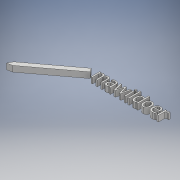
# Autodesk Inventor part: Matt
Saved by Autodesk Inventor 2017 (Build 210142000, 142)
## iProperties
Created: 2021-02-26
Part Number: Matt
Material: Generic
Document SubType Name: Modeling
Designer: paulg
Density: 1 g/cm^3
Appearance: Default
Author: paulg
Autodesk Inventor part; units mm, degrees
ref_plane "YZ Plane" through (0, 0, 0) normal (1, 0, 0) x (0, 1, 0)
ref_plane "XZ Plane" through (0, 0, 0) normal (0, 1, 0) x (-1, 0, 0)
ref_plane "XY Plane" through (0, 0, 0) normal (0, 0, 1) x (1, 0, 0)
sketch "Sketch1" plane through (0, 0, 0) normal (0, 0, 1) x (1, 0, 0)
  line L0 (-0.0217, 0.1086) -> (95.9171, 0.1086) construction
  line L1 (95.9171, 0.1086) -> (95.9171, -3.6211) construction
  line L2 (95.9171, -3.6211) -> (-0.0217, -3.6211) construction
  line L3 (-0.0217, -3.6211) -> (-0.0217, 0.1086) construction
  line L4 (-41.7116, -36.1087) -> (-2.9577, -7.16)
  line L5 (-2.9577, -7.16) -> (-5.3043, -4.0186)
  line L6 (-5.3043, -4.0186) -> (-44.0582, -32.9673)
  line L7 (-44.0582, -32.9673) -> (-41.7116, -36.1087)
  line L8 (-41.7116, -36.1087) -> (-5.3043, -4.0186) construction
  line L9 (-2.9577, -7.16) -> (-44.0582, -32.9673) construction
  line L10 (-44.0582, -32.9673) -> (-46.1916, -37.008)
  line L11 (-46.1916, -37.008) -> (-41.7116, -36.1087)
  line L12 (-46.1916, -37.008) -> (-42.8849, -34.538) construction
  line L13 (9.4029, -10.3371) -> (9.4029, -5.9935)
  spline S0 degree 2 poles (9.4029, -5.9935) (9.4029, -5.4748) (9.3219, -4.5915) (9.1922, -4.3484) knots 0 0 0 1 2 2 2
  spline S1 degree 2 poles (9.1922, -4.3484) (9.0625, -4.081) (8.5682, -3.8217) (8.1387, -3.8217) knots 0 0 0 1 2 2 2
  spline S2 degree 2 poles (8.1387, -3.8217) (7.7497, -3.8217) (6.8583, -4.2998) (6.3883, -4.7536) knots 0 0 0 1 2 2 2
  spline S3 degree 2 poles (6.3883, -4.7536) (6.3964, -4.867) (6.4126, -5.1831) (6.4126, -5.3938) knots 0 0 0 1 2 2 2
  line L14 (6.4126, -5.3938) -> (6.4126, -10.3371)
  line L15 (6.4126, -10.3371) -> (5.1484, -10.3371)
  line L16 (5.1484, -10.3371) -> (5.1484, -5.9935)
  spline S4 degree 2 poles (5.1484, -5.9935) (5.1484, -5.4748) (5.0674, -4.5915) (4.9378, -4.3484) knots 0 0 0 1 2 2 2
  spline S5 degree 2 poles (4.9378, -4.3484) (4.8081, -4.081) (4.3138, -3.8217) (3.8843, -3.8217) knots 0 0 0 1 2 2 2
  spline S6 degree 2 poles (3.8843, -3.8217) (3.4791, -3.8217) (2.5796, -4.3322) (2.1582, -4.7293) knots 0 0 0 1 2 2 2
  line L17 (2.1582, -4.7293) -> (2.1582, -10.3371)
  line L18 (2.1582, -10.3371) -> (0.894, -10.3371)
  line L19 (0.894, -10.3371) -> (0.894, -2.833)
  line L20 (0.894, -2.833) -> (2.1582, -2.833)
  line L21 (2.1582, -2.833) -> (2.1582, -3.6596)
  spline S7 degree 2 poles (2.1582, -3.6596) (2.6525, -3.1653) (3.6249, -2.6223) (4.2084, -2.6223) knots 0 0 0 1 2 2 2
  spline S8 degree 2 poles (4.2084, -2.6223) (4.8729, -2.6223) (5.9021, -3.2301) (6.1695, -3.9189) knots 0 0 0 1 2 2 2
  spline S9 degree 2 poles (6.1695, -3.9189) (6.7449, -3.2787) (7.8308, -2.6223) (8.4629, -2.6223) knots 0 0 0 1 2 2 2
  spline S10 degree 2 poles (8.4629, -2.6223) (8.9491, -2.6223) (9.7433, -2.9221) (10.035, -3.2625) knots 0 0 0 1 2 2 2
  spline S11 degree 2 poles (10.035, -3.2625) (10.3348, -3.6029) (10.6671, -4.6239) (10.6671, -5.3938) knots 0 0 0 1 2 2 2
  line L22 (10.6671, -5.3938) -> (10.6671, -10.3371)
  line L23 (10.6671, -10.3371) -> (9.4029, -10.3371)
  spline S12 degree 2 poles (16.6233, -9.5429) (16.4694, -9.6563) (15.9507, -10.0615) (15.7076, -10.1831) knots 0 0 0 1 2 2 2
  spline S13 degree 2 poles (15.7076, -10.1831) (15.3754, -10.3614) (14.7514, -10.5478) (14.1841, -10.5478) knots 0 0 0 1 2 2 2
  spline S14 degree 2 poles (14.1841, -10.5478) (13.7222, -10.5478) (12.8875, -10.1993) (12.5715, -9.8833) knots 0 0 0 1 2 2 2
  spline S15 degree 2 poles (12.5715, -9.8833) (12.2716, -9.5753) (11.907, -8.6677) (11.907, -8.1653) knots 0 0 0 1 2 2 2
  spline S16 degree 2 poles (11.907, -8.1653) (11.907, -7.3873) (12.5634, -6.2852) (13.2765, -5.9692) knots 0 0 0 1 2 2 2
  spline S17 degree 2 poles (13.2765, -5.9692) (13.9086, -5.6774) (15.6266, -5.4586) (16.6233, -5.4019) knots 0 0 0 1 2 2 2
  line L24 (16.6233, -5.4019) -> (16.6233, -5.1588)
  spline S18 degree 2 poles (16.6233, -5.1588) (16.6233, -4.7212) (16.3559, -4.1782) (16.1128, -4.0243) knots 0 0 0 1 2 2 2
  spline S19 degree 2 poles (16.1128, -4.0243) (15.8697, -3.8703) (15.1728, -3.773) (14.8, -3.773) knots 0 0 0 1 2 2 2
  spline S20 degree 2 poles (14.8, -3.773) (14.3624, -3.773) (13.1792, -4.0324) (12.5877, -4.2836) knots 0 0 0 1 2 2 2
  line L25 (12.5877, -4.2836) -> (12.5147, -4.2836)
  line L26 (12.5147, -4.2836) -> (12.5147, -2.9951)
  spline S21 degree 2 poles (12.5147, -2.9951) (12.8632, -2.8978) (14.1679, -2.6547) (14.8081, -2.6547) knots 0 0 0 1 2 2 2
  spline S22 degree 2 poles (14.8081, -2.6547) (15.5861, -2.6547) (16.6476, -2.8978) (17.069, -3.2139) knots 0 0 0 1 2 2 2
  spline S23 degree 2 poles (17.069, -3.2139) (17.4823, -3.5218) (17.8875, -4.5024) (17.8875, -5.2074) knots 0 0 0 1 2 2 2
  line L27 (17.8875, -5.2074) -> (17.8875, -10.3371)
  line L28 (17.8875, -10.3371) -> (16.6233, -10.3371)
  line L29 (16.6233, -10.3371) -> (16.6233, -9.5429)
  line L30 (16.6233, -8.4894) -> (16.6233, -6.4068)
  spline S24 degree 2 poles (16.6233, -6.4068) (16.1695, -6.4473) (14.8, -6.585) (14.3705, -6.7147) knots 0 0 0 1 2 2 2
  spline S25 degree 2 poles (14.3705, -6.7147) (13.8681, -6.8687) (13.2117, -7.5089) (13.2117, -8.0761) knots 0 0 0 1 2 2 2
  spline S26 degree 2 poles (13.2117, -8.0761) (13.2117, -8.7244) (13.941, -9.3808) (14.6379, -9.3808) knots 0 0 0 1 2 2 2
  spline S27 degree 2 poles (14.6379, -9.3808) (15.2295, -9.3808) (16.2019, -8.8703) (16.6233, -8.4894) knots 0 0 0 1 2 2 2
  line L31 (28.7546, -2.833) -> (26.8502, -10.3371)
  line L32 (26.8502, -10.3371) -> (25.6833, -10.3371)
  line L33 (25.6833, -10.3371) -> (23.8519, -4.551)
  line L34 (23.8519, -4.551) -> (22.0285, -10.3371)
  line L35 (22.0285, -10.3371) -> (20.8697, -10.3371)
  line L36 (20.8697, -10.3371) -> (18.9491, -2.833)
  line L37 (18.9491, -2.833) -> (20.2619, -2.833)
  line L38 (20.2619, -2.833) -> (21.5909, -8.6434)
  line L39 (21.5909, -8.6434) -> (23.3656, -2.833)
  line L40 (23.3656, -2.833) -> (24.411, -2.833)
  line L41 (24.411, -2.833) -> (26.2343, -8.6434)
  line L42 (26.2343, -8.6434) -> (27.4823, -2.833)
  line L43 (27.4823, -2.833) -> (28.7546, -2.833)
  line L44 (31.1533, -10.3371) -> (29.8891, -10.3371)
  line L45 (29.8891, -10.3371) -> (29.8891, -2.833)
  line L46 (29.8891, -2.833) -> (31.1533, -2.833)
  line L47 (31.1533, -2.833) -> (31.1533, -10.3371)
  line L48 (31.2425, -1.585) -> (29.8081, -1.585)
  line L49 (29.8081, -1.585) -> (29.8081, -0.2722)
  line L50 (29.8081, -0.2722) -> (31.2425, -0.2722)
  line L51 (31.2425, -0.2722) -> (31.2425, -1.585)
  line L52 (34.2976, -10.3371) -> (33.0334, -10.3371)
  line L53 (33.0334, -10.3371) -> (33.0334, 0.1086)
  line L54 (33.0334, 0.1086) -> (34.2976, 0.1086)
  line L55 (34.2976, 0.1086) -> (34.2976, -10.3371)
  line L56 (41.9232, -10.3371) -> (40.659, -10.3371)
  line L57 (40.659, -10.3371) -> (40.659, -9.5753)
  spline S28 degree 2 poles (40.659, -9.5753) (40.3672, -9.8184) (39.9378, -10.1426) (39.646, -10.2803) knots 0 0 0 1 2 2 2
  spline S29 degree 2 poles (39.646, -10.2803) (39.3786, -10.41) (38.8032, -10.5478) (38.4224, -10.5478) knots 0 0 0 1 2 2 2
  spline S30 degree 2 poles (38.4224, -10.5478) (37.8065, -10.5478) (36.7692, -10.0372) (36.4045, -9.5429) knots 0 0 0 1 2 2 2
  spline S31 degree 2 poles (36.4045, -9.5429) (36.0399, -9.0486) (35.6347, -7.5899) (35.6347, -6.6418) knots 0 0 0 1 2 2 2
  spline S32 degree 2 poles (35.6347, -6.6418) (35.6347, -5.6531) (36.1452, -4.2106) (36.5909, -3.6677) knots 0 0 0 1 2 2 2
  spline S33 degree 2 poles (36.5909, -3.6677) (37.0042, -3.1815) (38.163, -2.6223) (38.8032, -2.6223) knots 0 0 0 1 2 2 2
  spline S34 degree 2 poles (38.8032, -2.6223) (39.3624, -2.6223) (40.1971, -2.8735) (40.659, -3.1328) knots 0 0 0 1 2 2 2
  line L58 (40.659, -3.1328) -> (40.659, 0.1086)
  line L59 (40.659, 0.1086) -> (41.9232, 0.1086)
  line L60 (41.9232, 0.1086) -> (41.9232, -10.3371)
  line L61 (40.659, -8.5137) -> (40.659, -4.1782)
  spline S35 degree 2 poles (40.659, -4.1782) (40.189, -3.9513) (39.4434, -3.7811) (39.0139, -3.7811) knots 0 0 0 1 2 2 2
  spline S36 degree 2 poles (39.0139, -3.7811) (38.0415, -3.7811) (36.9394, -5.2398) (36.9394, -6.6174) knots 0 0 0 1 2 2 2
  spline S37 degree 2 poles (36.9394, -6.6174) (36.9394, -7.9465) (37.7822, -9.3484) (38.7141, -9.3484) knots 0 0 0 1 2 2 2
  spline S38 degree 2 poles (38.7141, -9.3484) (39.2084, -9.3484) (40.2133, -8.8946) (40.659, -8.5137) knots 0 0 0 1 2 2 2
  spline S39 degree 2 poles (49.9215, -6.585) (49.9215, -8.4813) (48.0982, -10.5478) (46.5747, -10.5478) knots 0 0 0 1 2 2 2
  spline S40 degree 2 poles (46.5747, -10.5478) (45.0107, -10.5478) (43.2198, -8.4165) (43.2198, -6.585) knots 0 0 0 1 2 2 2
  spline S41 degree 2 poles (43.2198, -6.585) (43.2198, -4.705) (45.0674, -2.6223) (46.5747, -2.6223) knots 0 0 0 1 2 2 2
  spline S42 degree 2 poles (46.5747, -2.6223) (48.0982, -2.6223) (49.9215, -4.6969) (49.9215, -6.585) knots 0 0 0 1 2 2 2
  spline S43 degree 2 poles (48.6168, -6.585) (48.6168, -5.1264) (47.5553, -3.7082) (46.5747, -3.7082) knots 0 0 0 1 2 2 2
  spline S44 degree 2 poles (46.5747, -3.7082) (45.5942, -3.7082) (44.5245, -5.1264) (44.5245, -6.585) knots 0 0 0 1 2 2 2
  spline S45 degree 2 poles (44.5245, -6.585) (44.5245, -8.0032) (45.5942, -9.4619) (46.5747, -9.4619) knots 0 0 0 1 2 2 2
  spline S46 degree 2 poles (46.5747, -9.4619) (47.5472, -9.4619) (48.6168, -8.0275) (48.6168, -6.585) knots 0 0 0 1 2 2 2
  spline S47 degree 2 poles (54.4758, -10.5072) (52.6768, -10.5072) (50.6995, -8.4894) (50.6995, -6.6256) knots 0 0 0 1 2 2 2
  spline S48 degree 2 poles (50.6995, -6.6256) (50.6995, -4.7941) (52.6201, -2.6223) (54.1679, -2.6223) knots 0 0 0 1 2 2 2
  spline S49 degree 2 poles (54.1679, -2.6223) (54.8648, -2.6223) (55.9426, -3.0275) (56.3397, -3.457) knots 0 0 0 1 2 2 2
  spline S50 degree 2 poles (56.3397, -3.457) (56.7449, -3.8865) (57.1744, -5.1264) (57.1744, -6.0259) knots 0 0 0 1 2 2 2
  line L62 (57.1744, -6.0259) -> (57.1744, -6.7147)
  line L63 (57.1744, -6.7147) -> (51.9799, -6.7147)
  spline S51 degree 2 poles (51.9799, -6.7147) (51.9799, -8.0194) (53.2927, -9.4051) (54.4596, -9.4051) knots 0 0 0 1 2 2 2
  spline S52 degree 2 poles (54.4596, -9.4051) (54.8729, -9.4051) (55.6752, -9.2187) (55.9993, -9.0729) knots 0 0 0 1 2 2 2
  spline S53 degree 2 poles (55.9993, -9.0729) (56.3397, -8.9108) (56.8097, -8.6272) (56.9637, -8.4975) knots 0 0 0 1 2 2 2
  line L64 (56.9637, -8.4975) -> (57.0366, -8.4975)
  line L65 (57.0366, -8.4975) -> (57.0366, -9.8751)
  spline S54 degree 2 poles (57.0366, -9.8751) (56.8178, -9.9643) (56.1533, -10.2236) (55.894, -10.2965) knots 0 0 0 1 2 2 2
  spline S55 degree 2 poles (55.894, -10.2965) (55.5293, -10.4019) (54.9296, -10.5072) (54.4758, -10.5072) knots 0 0 0 1 2 2 2
  spline S56 degree 2 poles (55.9426, -5.7503) (55.9264, -5.2398) (55.7157, -4.4943) (55.5131, -4.2431) knots 0 0 0 1 2 2 2
  spline S57 degree 2 poles (55.5131, -4.2431) (55.2943, -3.9594) (54.6055, -3.6596) (54.095, -3.6596) knots 0 0 0 1 2 2 2
  spline S58 degree 2 poles (54.095, -3.6596) (53.5925, -3.6596) (52.8875, -3.9594) (52.5958, -4.2512) knots 0 0 0 1 2 2 2
  spline S59 degree 2 poles (52.5958, -4.2512) (52.3121, -4.551) (52.0204, -5.2722) (51.9799, -5.7503) knots 0 0 0 1 2 2 2
  line L66 (51.9799, -5.7503) -> (55.9426, -5.7503)
  line L67 (62.4337, -4.1863) -> (62.3689, -4.1863)
  spline S60 degree 2 poles (62.3689, -4.1863) (62.223, -4.1458) (61.907, -4.1296) (61.6882, -4.1296) knots 0 0 0 1 2 2 2
  spline S61 degree 2 poles (61.6882, -4.1296) (61.1776, -4.1296) (60.1728, -4.5753) (59.719, -5.0129) knots 0 0 0 1 2 2 2
  line L68 (59.719, -5.0129) -> (59.719, -10.3371)
  line L69 (59.719, -10.3371) -> (58.4548, -10.3371)
  line L70 (58.4548, -10.3371) -> (58.4548, -2.833)
  line L71 (58.4548, -2.833) -> (59.719, -2.833)
  line L72 (59.719, -2.833) -> (59.719, -3.9513)
  spline S62 degree 2 poles (59.719, -3.9513) (60.4078, -3.3354) (61.4369, -2.833) (61.9232, -2.833) knots 0 0 0 1 2 2 2
  spline S63 degree 2 poles (61.9232, -2.833) (62.1177, -2.833) (62.3121, -2.8492) (62.4337, -2.8735) knots 0 0 0 1 2 2 2
  line L73 (62.4337, -2.8735) -> (62.4337, -4.1863)
  point P0 (0, 0)
  point P1 (-23.5079, -20.0636)
  constraints: 18 end point, 3 midpoint, 3 parallel, 1 perpendicular, 2 other
extrude "Extrusion1" add sketch "Sketch1" along normal blind 5
body "Solid1"
